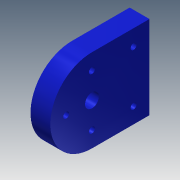
# Autodesk Inventor part: komatex2
Saved by Autodesk Inventor 2013 (Build 170138000, 138)
## iProperties
Created: 2013-01-31
Part Number: komatex2
Material: Generic
Document SubType Name: Modeling
Designer: idle-rug
Density: 1 g/cm^3
Author: idle-rug
Autodesk Inventor part; units mm, degrees
ref_plane "YZ Plane" through (0, 0, 0) normal (1, 0, 0) x (0, 1, 0)
ref_plane "XZ Plane" through (0, 0, 0) normal (0, 1, 0) x (-1, 0, 0)
ref_plane "XY Plane" through (0, 0, 0) normal (0, 0, 1) x (1, 0, 0)
sketch "Sketch1" plane through (0, 0, 0) normal (1, 0, 0) x (0, 1, 0)
  circle A0 centre (6.5, 13) radius 1.5
  circle A1 centre (-14.5, 13) radius 1.5
  circle A2 centre (-27.5, 0) radius 1.5
  circle A3 centre (-14.5, -13) radius 1.5
  circle A4 centre (6.5, -13) radius 1.5
  circle A5 centre (-14.5, 0) radius 3.5
  arc A6 (-14.5, 21) -> (-14.5, -21) centre (-14.5, 0) ccw
  line L0 (-14.5, -21) -> (14.5, -21)
  line L1 (14.5, -21) -> (14.5, 21)
  line L2 (14.5, 21) -> (-14.5, 21)
  point P0 (0, 0)
  point P1 (0, 0)
  constraints: 7 centre point, 6 end point, 2 point on circle
extrude "Extrusion1" add sketch "Sketch1" along normal blind 17
sketch "Sketch2" plane through (17, 0, 0) normal (1, 0, 0) x (0, 0, -1)
  circle A0 centre (0, -14.5) radius 3.5 projected
  circle A1 centre (13, 6.5) radius 1.5 projected
  circle A2 centre (13, -14.5) radius 1.5 projected
  circle A3 centre (0, -27.5) radius 1.5 projected
  circle A4 centre (-13, -14.5) radius 1.5 projected
  circle A5 centre (-13, 6.5) radius 1.5 projected
  arc A6 (-21, -14.5) -> (21, -14.5) centre (0, -14.5) ccw projected
  line L0 (21, -14.5) -> (21, 14.5) projected
  line L1 (21, 14.5) -> (-21, 14.5) projected
  line L2 (-21, 14.5) -> (-21, -14.5) projected
  point P0 (0, 0)
extrude "Extrusion2" cut sketch "Sketch2" against normal blind 4
sketch "Sketch3" plane through (13, 0, 0) normal (1, 0, 0) x (0, 0, -1)
  circle A0 centre (0, -14.5) radius 3.5 projected
  circle A1 centre (-13, 6.5) radius 1.5 projected
  circle A2 centre (-13, -14.5) radius 1.5 projected
  circle A3 centre (0, -27.5) radius 1.5 projected
  circle A4 centre (13, -14.5) radius 1.5 projected
  circle A5 centre (13, 6.5) radius 1.5 projected
  arc A6 (-21, -14.5) -> (21, -14.5) centre (0, -14.5) ccw projected
  line L0 (21, 14.5) -> (21, -14.5) projected
  line L1 (-21, 14.5) -> (21, 14.5) projected
  line L2 (-21, -14.5) -> (-21, 14.5) projected
  point P0 (0, 0)
extrude "Extrusion3" cut sketch "Sketch3" against normal blind 3
body "Solid1"
